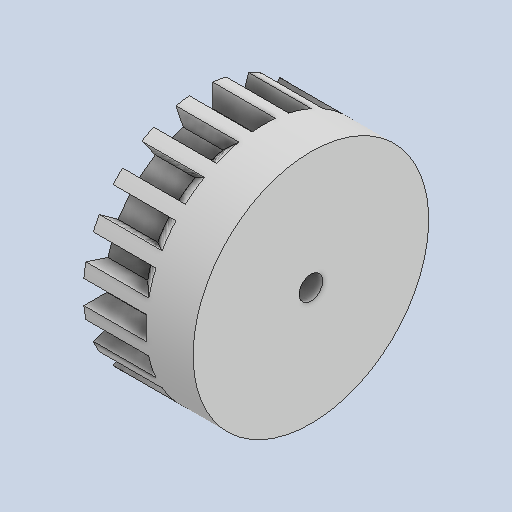
# Autodesk Inventor part: koło_minisumo
Saved by Autodesk Inventor 2023 (Build 270158000, 158)
## iProperties
Created: 2022-10-10
Part Number: koło_minisumo
Material: Generic
Document SubType Name: Modeling
Designer: komputer
Density: 1 g/cm^3
Appearance: Default
Author: komputer
Autodesk Inventor part; units mm, degrees
ref_plane "YZ Plane" through (0, 0, 0) normal (1, 0, 0) x (0, 1, 0)
ref_plane "XZ Plane" through (0, 0, 0) normal (0, 1, 0) x (-1, 0, 0)
ref_plane "XY Plane" through (0, 0, 0) normal (0, 0, 1) x (1, 0, 0)
sketch "Sketch1" plane through (0, 0, 0) normal (1, 0, 0) x (0, 1, 0)
  circle A0 centre (0, 0) radius 15.02
  dimension "d0" = 30.04
  constraints: 1 centre point, 1 coincident
  measures "d0" diameter of A0
extrude "Extrusion1" add sketch "Sketch1" along normal blind 14
sketch "Sketch2" plane through (14, 0, 0) normal (1, 0, 0) x (0, 0, -1)
  circle A0 centre (0, 0) radius 1.5
  dimension "d3" = 3
  constraints: 1 centre point, 1 coincident
  measures "d3" diameter of A0
extrude "Extrusion2" cut sketch "Sketch2" against normal blind 10
sketch "Sketch3" plane through (0, 0, 0) normal (-1, 0, 0) x (0, 0, 1)
  circle A0 centre (0, 0) radius 1.5
  circle A1 centre (0, 0) radius 11.001815
  circle A2 centre (0, 0) radius 15.02
  line L0 (-15.02, 0) -> (-11.994991, 0)
  line L1 (-11.994991, 0) -> (-11.994991, 1.5)
  line L2 (-11.994991, 1.5) -> (-19.829964, 1.5)
  line L3 (-11.994991, 0) -> (-11.994991, -1.5)
  line L4 (-11.994991, -1.5) -> (-19.829964, -1.5)
  line L5 (-19.829964, -1.5) -> (-19.829964, 1.5)
  line L6 (-10.944389, -5.133241) -> (-18.395891, -7.554381)
  line L7 (-11.87144, -2.280071) -> (-19.322942, -4.701211)
  line L8 (-11.407914, -3.706656) -> (-10.944389, -5.133241)
  line L9 (-11.407914, -3.706656) -> (-11.87144, -2.280071)
  line L10 (-18.395891, -7.554381) -> (-19.322942, -4.701211)
  line L11 (-8.822473, -8.264004) -> (-15.1611, -12.869286)
  line L12 (-10.585829, -5.836953) -> (-16.924456, -10.442235)
  line L13 (-9.704151, -7.050479) -> (-8.822473, -8.264004)
  line L14 (-9.704151, -7.050479) -> (-10.585829, -5.836953)
  line L15 (-15.1611, -12.869286) -> (-16.924456, -10.442235)
  line L16 (-5.836953, -10.585829) -> (-10.442235, -16.924456)
  line L17 (-8.264004, -8.822473) -> (-12.869286, -15.1611)
  line L18 (-7.050479, -9.704151) -> (-5.836953, -10.585829)
  line L19 (-7.050479, -9.704151) -> (-8.264004, -8.822473)
  line L20 (-10.442235, -16.924456) -> (-12.869286, -15.1611)
  line L21 (-2.280071, -11.87144) -> (-4.701211, -19.322942)
  line L22 (-5.133241, -10.944389) -> (-7.554381, -18.395891)
  line L23 (-3.706656, -11.407914) -> (-2.280071, -11.87144)
  line L24 (-3.706656, -11.407914) -> (-5.133241, -10.944389)
  line L25 (-4.701211, -19.322942) -> (-7.554381, -18.395891)
  line L26 (1.5, -11.994991) -> (1.5, -19.829964)
  line L27 (-1.5, -11.994991) -> (-1.5, -19.829964)
  line L28 (0, -11.994991) -> (1.5, -11.994991)
  line L29 (0, -11.994991) -> (-1.5, -11.994991)
  line L30 (1.5, -19.829964) -> (-1.5, -19.829964)
  line L31 (5.133241, -10.944389) -> (7.554381, -18.395891)
  line L32 (2.280071, -11.87144) -> (4.701211, -19.322942)
  line L33 (3.706656, -11.407914) -> (5.133241, -10.944389)
  line L34 (3.706656, -11.407914) -> (2.280071, -11.87144)
  line L35 (7.554381, -18.395891) -> (4.701211, -19.322942)
  line L36 (8.264004, -8.822473) -> (12.869286, -15.1611)
  line L37 (5.836953, -10.585829) -> (10.442235, -16.924456)
  line L38 (7.050479, -9.704151) -> (8.264004, -8.822473)
  line L39 (7.050479, -9.704151) -> (5.836953, -10.585829)
  line L40 (12.869286, -15.1611) -> (10.442235, -16.924456)
  line L41 (10.585829, -5.836953) -> (16.924456, -10.442235)
  line L42 (8.822473, -8.264004) -> (15.1611, -12.869286)
  line L43 (9.704151, -7.050479) -> (10.585829, -5.836953)
  line L44 (9.704151, -7.050479) -> (8.822473, -8.264004)
  line L45 (16.924456, -10.442235) -> (15.1611, -12.869286)
  line L46 (11.87144, -2.280071) -> (19.322942, -4.701211)
  line L47 (10.944389, -5.133241) -> (18.395891, -7.554381)
  line L48 (11.407914, -3.706656) -> (11.87144, -2.280071)
  line L49 (11.407914, -3.706656) -> (10.944389, -5.133241)
  line L50 (19.322942, -4.701211) -> (18.395891, -7.554381)
  line L51 (11.994991, 1.5) -> (19.829964, 1.5)
  line L52 (11.994991, -1.5) -> (19.829964, -1.5)
  line L53 (11.994991, 0) -> (11.994991, 1.5)
  line L54 (11.994991, 0) -> (11.994991, -1.5)
  line L55 (19.829964, 1.5) -> (19.829964, -1.5)
  line L56 (10.944389, 5.133241) -> (18.395891, 7.554381)
  line L57 (11.87144, 2.280071) -> (19.322942, 4.701211)
  line L58 (11.407914, 3.706656) -> (10.944389, 5.133241)
  line L59 (11.407914, 3.706656) -> (11.87144, 2.280071)
  line L60 (18.395891, 7.554381) -> (19.322942, 4.701211)
  line L61 (8.822473, 8.264004) -> (15.1611, 12.869286)
  line L62 (10.585829, 5.836953) -> (16.924456, 10.442235)
  line L63 (9.704151, 7.050479) -> (8.822473, 8.264004)
  line L64 (9.704151, 7.050479) -> (10.585829, 5.836953)
  line L65 (15.1611, 12.869286) -> (16.924456, 10.442235)
  line L66 (5.836953, 10.585829) -> (10.442235, 16.924456)
  line L67 (8.264004, 8.822473) -> (12.869286, 15.1611)
  line L68 (7.050479, 9.704151) -> (5.836953, 10.585829)
  line L69 (7.050479, 9.704151) -> (8.264004, 8.822473)
  line L70 (10.442235, 16.924456) -> (12.869286, 15.1611)
  line L71 (2.280071, 11.87144) -> (4.701211, 19.322942)
  line L72 (5.133241, 10.944389) -> (7.554381, 18.395891)
  line L73 (3.706656, 11.407914) -> (2.280071, 11.87144)
  line L74 (3.706656, 11.407914) -> (5.133241, 10.944389)
  line L75 (4.701211, 19.322942) -> (7.554381, 18.395891)
  line L76 (-1.5, 11.994991) -> (-1.5, 19.829964)
  line L77 (1.5, 11.994991) -> (1.5, 19.829964)
  line L78 (0, 11.994991) -> (-1.5, 11.994991)
  line L79 (0, 11.994991) -> (1.5, 11.994991)
  line L80 (-1.5, 19.829964) -> (1.5, 19.829964)
  line L81 (-5.133241, 10.944389) -> (-7.554381, 18.395891)
  line L82 (-2.280071, 11.87144) -> (-4.701211, 19.322942)
  line L83 (-3.706656, 11.407914) -> (-5.133241, 10.944389)
  line L84 (-3.706656, 11.407914) -> (-2.280071, 11.87144)
  line L85 (-7.554381, 18.395891) -> (-4.701211, 19.322942)
  line L86 (-8.264004, 8.822473) -> (-12.869286, 15.1611)
  line L87 (-5.836953, 10.585829) -> (-10.442235, 16.924456)
  line L88 (-7.050479, 9.704151) -> (-8.264004, 8.822473)
  line L89 (-7.050479, 9.704151) -> (-5.836953, 10.585829)
  line L90 (-12.869286, 15.1611) -> (-10.442235, 16.924456)
  line L91 (-10.585829, 5.836953) -> (-16.924456, 10.442235)
  line L92 (-8.822473, 8.264004) -> (-15.1611, 12.869286)
  line L93 (-9.704151, 7.050479) -> (-10.585829, 5.836953)
  line L94 (-9.704151, 7.050479) -> (-8.822473, 8.264004)
  line L95 (-16.924456, 10.442235) -> (-15.1611, 12.869286)
  line L96 (-11.87144, 2.280071) -> (-19.322942, 4.701211)
  line L97 (-10.944389, 5.133241) -> (-18.395891, 7.554381)
  line L98 (-11.407914, 3.706656) -> (-11.87144, 2.280071)
  line L99 (-11.407914, 3.706656) -> (-10.944389, 5.133241)
  line L100 (-19.322942, 4.701211) -> (-18.395891, 7.554381)
  point P0 (-1.5, -14.944912)
  point P1 (1.5, -14.944912)
  point P2 (-6.044817, -13.749931)
  point P3 (-3.191647, -14.676982)
  point P4 (-9.997924, -11.20901)
  point P5 (-7.570873, -12.972366)
  dimension "d8" = 360
  constraints: 202 end point, 4 perpendicular, 1 centre point, 1 coincident, 1 horizontal, 1 vertical, 203 other
extrude "Extrusion3" cut sketch "Sketch3" against normal blind 5 contours A2 L52 L54 L53 L51 | A2 L51 L55 L52 | L57 L59 L58 L56 A2 | A2 L56 L60 L57 | L46 L50 L47 A2 | A2 L47 L49 L48 L46 | L62 L64 L63 L61 A2 | A2 L61 L65 L62 | L41 L45 L42 A2 | A2 L42 L44 L43 L41 | L67 L69 L68 L66 A2 | A2 L66 L70 L67 | L36 L40 L37 A2 | A2 L37 L39 L38 L36 | L72 L74 L73 L71 A2 | A2 L71 L75 L72 | L31 L35 L32 A2 | A2 L32 L34 L33 L31 | L77 L79 L78 L76 A2 | A2 L76 L80 L77 | A2 L27 L29 L28 L26 | L82 L84 L83 L81 A2 | A2 L81 L85 L82 | A2 L22 L24 L23 L21 | L87 L89 L88 L86 A2 | A2 L86 L90 L87 | A2 L17 L19 L18 L16 | L92 L94 L93 L91 A2 | A2 L91 L95 L92 | L11 L15 L12 A2 | A2 L12 L14 L13 L11 | L97 L99 L98 L96 A2 | A2 L96 L100 L97 | L6 L10 L7 A2 | A2 L7 L9 L8 L6 | L2 L1 L0 A2 | A2 L4 L5 L2 | A2 L0 L3 L4
chamfer "Chamfer1" distance 3 angle 45 21 edges at (5, 14.2849, -4.6414) (5, 15.0012, 0.7509) (5, 15.0012, -0.7509) (5, 14.2849, 4.6414) (5, 12.1514, 8.8285) (5, 8.8285, 12.1514) (5, 4.6414, 14.2849) (5, 0, 15.02) (5, -4.6414, 14.2849) (5, -8.8285, 12.1514) (5, -12.1514, 8.8285) (5, -14.2849, 4.6414) (5, -15.02, 0) (5, -14.2849, -4.6414) (5, -12.1514, -8.8285) (5, -8.8285, -12.1514) (5, -4.6414, -14.2849) (5, 0, -15.02) (5, 4.6414, -14.2849) (5, 8.8285, -12.1514) (5, 12.1514, -8.8285)
sketch "Sketch4" plane through (0, 0, 0) normal (-1, 0, 0) x (0, 0, 1)
  circle A0 centre (0, 0) radius 8.984873
  constraints: 1 centre point, 1 coincident
extrude "Extrusion4" cut sketch "Sketch4" against normal blind 2
body "Solid1"
